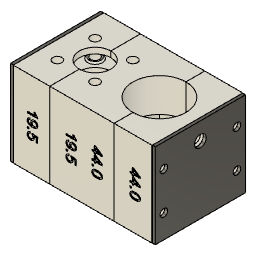
E39steerModuleCase v1 (Autodesk Fusion 360 design; units mm, degrees)
Autodesk Fusion 360 part; units mm, degrees
note: some values were not read from the file. Set by a fixed rule: which face or edge a step refers to.
sketch "Sketch1" plane through (0, 0, 0) normal (0, 0, 1) x (1, 0, 0)
  circle A0 centre (0, 0) radius 9.75
  line L0 (0, 0) -> (-27.3416, 27.3416) construction
  line L1 (0, 0) -> (-38.1238, 0) construction
  circle A1 centre (-12.9047, 12.9047) radius 9.3
  line L2 (0, 0) -> (-25, 0)
  line L3 (-25, 0) -> (-25, 31)
  line L4 (-25, 31) -> (0, 31)
  line L5 (0, 31) -> (0, 0)
  circle A2 centre (-12.9047, 12.9047) radius 3.1
  circle A3 centre (0, 0) radius 10.75
  circle A4 centre (-12.9047, 12.9047) radius 4
  line L6 (0, 31) -> (0, 19.6239) construction
  line L7 (-25, 0) -> (-19.6239, 0) construction
  circle A5 centre (-12.9047, 12.9047) radius 8.5 construction
  circle A6 centre (-12.9047, 12.9047) radius 2
  line L8 (-12.9047, 22.2047) -> (0, 22.2047)
  line L9 (-22.2047, 12.9047) -> (-22.2047, 0)
  dimension "d1" = 19.5
  dimension "d3" = 45
  dimension "d4" = 18.6
  dimension "d6" = 31
  dimension "d7" = 6.2
  dimension "d8" = 21.5
  dimension "d15" = 8
  dimension "d119" = 17
  dimension "d151" = 4
  dimension "d172" = 18.25
  dimension "d173" = 25
  constraint coincident A0.centre L0.start
  constraint horizontal L1
  constraint horizontal L2
  constraint vertical L3
  constraint horizontal L4
  constraint vertical L5
  constraint concentric A1 A2
  constraint concentric A2 A4
  constraint perpendicular L4 L6
  constraint perpendicular L3 L7
  constraint concentric A4 A5
  constraint concentric A2 A6
  constraint coincident A1 L8.start
  constraint coincident L5 L8.end
  constraint tangent A1 L8
  constraint perpendicular L5 L8
  constraint vertical L9
  constraint coincident A1 L9.start
  constraint coincident L1 L9.end
  measures "d1" diameter of A0
  measures "d3" angle of L0 L1
  measures "d4" diameter of A1
  measures "d6" distance of A0.centre L4.end
  measures "d7" diameter of A2
  measures "d8" diameter of A3
  measures "d15" diameter of A4
  measures "d119" diameter of A5
  measures "d151" diameter of A6
  measures "d172" distance of A0.centre A1.centre
  measures "d173" distance of L3.end L4.end
extrude "Extrude1" add sketch "Sketch1" along normal blind 16 contours A1 L5 A3 L8 | A1 L2 A3 L9 | A1 A3 | A1 L2 L3 L4 L5 L8 L9 | A2 | A4 | A6 makes body 1
extrude "Extrude3" cut sketch "Sketch1" along normal blind 12 contours A0 A1 | A0 A1 A3 | A1 L5 A3 L8 | A1 L2 A3 L9 | A1 A3 | A4 bodies 1
extrude "Extrude2" cut sketch "Sketch1" along normal blind 14 contours A2 | A6 bodies 1
extrude "Extrude4" cut sketch "Sketch1" along normal blind 13 contours A4 bodies 1
extrude "Extrude15" add 1 faces at (-9.2311, 12.552, 13) along direction (0, 0, -1) blind 2 on bodies 1 bodies 1
extrude "Extrude20" add sketch "Sketch1" along normal blind 4 contours A1 L5 A3 L8 | A1 L2 A3 L9 | A1 A3 | A1 L2 L3 L4 L5 L8 L9 bodies 1
extrude "Extrude21" add sketch "Sketch1" along normal blind 5 contours A4 bodies 1
extrude "Extrude31" cut sketch "Sketch1" along normal up to surface (16 mm away) contours A6 bodies 1
chamfer "Chamfer2" distance 1 angle 45 2 edges at (-16.634, 11.4582, 12) (-16.634, 14.3512, 4) on bodies 1
ref_plane "WorkPlane2" through (-12.5, 15.5, -13) normal (0, 0, -1) x (-1, 0, 0)
mirror "Mirror1" about plane through (-12.5, 15.5, -13) normal (0, 0, -1) of bodies 1 makes body 2
extrude "Extrude5" cut 1 faces at (-10.1904, 12.6513, -40) along direction (0, 0, -1) blind 3 on bodies 2 bodies 2
extrude "Extrude6" add sketch "Sketch1" 1 faces at (-12.5577, 25.9987, 0) along normal up to surface contours A1 L5 A3 L8 | A1 L2 A3 L9 | A1 A3 | A1 L2 L3 L4 L5 L8 L9 end surface through (0, 0, -26) normal (0, 0, 1) offset 0 on bodies 1 bodies 1 2
sketch "Sketch3" plane through (-25, 0, 0) normal (-1, 0, 0) x (0, -1, 0)
  line L0 (0, -42) -> (0, 16)
  line L1 (0, 16) -> (-31, 16)
  line L2 (-31, 16) -> (-9.7868, 16) construction
  line L3 (-31, 16) -> (-25, 16) construction
  line L4 (-25, 16) -> (-25, 0) construction
  circle A0 centre (-25, 0) radius 2.6
  line L5 (-31, 16) -> (-31, -42)
  line L6 (-31, -42) -> (0, -42)
  circle A1 centre (-25, -26) radius 2.6
  dimension "d27" = 6
  dimension "d28" = 16
  dimension "d29" = 5.2
  dimension "d178" = 5.2
  dimension "d179" = 26
  constraint horizontal L2
  constraint coincident L1.end L2.start
  constraint perpendicular L3 L4
  constraint coincident L4.end A0.centre
  measures "d27" distance of L1.end L3.end
  measures "d28" distance of L3.end L4.end
  measures "d29" diameter of A0
  measures "d178" diameter of A1
  measures "d179" distance of L4.end A1.centre
extrude "Extrude7" cut sketch "Sketch3" against normal up to surface (25 mm away) contours A0 | A1 bodies 1
sketch "Sketch10" plane through (0, 0, 0) normal (1, 0, 0) x (0, 1, 0)
  circle A0 centre (25, 0) radius 2.6
  line L0 (22.2047, 4) -> (10.75, 4)
  line L1 (10.75, 4) -> (10.75, -30)
  line L2 (10.75, -30) -> (22.2047, -30)
  line L3 (22.2047, -38) -> (10.75, -38)
  line L4 (10.75, -38) -> (10.75, -42)
  line L5 (10.75, -42) -> (31, -42)
  line L6 (31, -42) -> (31, 16)
  line L7 (31, 16) -> (10.75, 16)
  line L8 (10.75, 16) -> (10.75, 12)
  line L9 (10.75, 12) -> (22.2047, 12)
  line L10 (10.75, 4) -> (10.75, -9) construction
  line L11 (22.25, -9) -> (26.25, -9)
  line L12 (26.25, -9) -> (26.25, -17)
  line L13 (26.25, -17) -> (22.25, -17)
  line L14 (22.25, -17) -> (22.25, -9)
  circle A1 centre (25, -26) radius 2.6
  line L15 (22.2047, 12) -> (22.2047, 4)
  line L16 (22.2047, -30) -> (22.2047, -38)
  dimension "d136" = 11.5
  dimension "d137" = 4
  dimension "d138" = 8
  dimension "d180" = 25
  constraint coincident L0.end L1.start
  constraint perpendicular L0 L10
  constraint horizontal L11
  constraint vertical L12
  constraint horizontal L13
  constraint vertical L14
  measures "d136" distance of L10.end L11.start
  measures "d137" distance of L11.start L11.end
  measures "d138" distance of L11.start L13.end
  measures "d180" distance of L7 L11.end
extrude "Extrude26" add sketch "Sketch10" along normal blind 5 contours L11 L12 L13 L14 bodies 1
mirror "Mirror2" about plane through (-10.75, 0, 0) normal (0, -1, 0) of bodies 1 merged
mirror "Mirror3" about plane through (0, -22.2047, 0) normal (1, 0, 0) of bodies 1 makes body 3
move_face "OffsetFaces1" offset -0.1 8 faces at (1.6667, 23.5833, -9) (1.6667, 26.25, -11.6667) (3.3333, 22.25, -14.3333) (1.6667, 24.9167, -17) (1.6667, -26.25, -11.6667) (1.6667, -24.9167, -17) (3.3333, -22.25, -14.3333) (1.6667, -23.5833, -9) on bodies 1
sketch "Sketch5" plane through (0, 0, -42) normal (0, 0, -1) x (1, 0, 0)
  circle A0 centre (12.9047, 12.9047) radius 3.1
  line L0 (0, -31) -> (25, -31)
  line L1 (25, 31) -> (0, 31)
  line L2 (0, 31) -> (0, 10.75)
  arc A1 (0, -10.75) -> (0, 10.75) centre (0, 0) ccw
  line L3 (0, -10.75) -> (0, -31)
  line L4 (24, 30.9926) -> (24, 30.9994) construction
  circle A2 centre (44, -0.0006) radius 18.1
  circle A3 centre (12.9047, -12.9047) radius 3.1
  line L5 (65, -21.1006) -> (23, -21.1006)
  line L6 (23, -21.1006) -> (23, 21.0994)
  line L7 (23, 21.0994) -> (65, 21.0994)
  line L8 (65, 21.0994) -> (65, -21.1006)
  line L9 (65, -21.1006) -> (23, 21.0994) construction
  line L10 (23, -21.1006) -> (65, 21.0994) construction
  point P0 (24, 9.8926)
  point P1 (24, -0.0006)
  point P2 (44, -0.0006)
  dimension "d126" = 36.2
  dimension "d182" = 44
  dimension "d183" = 42
  dimension "d184" = 42.2
  constraint horizontal L5
  constraint perpendicular L5 L6
  constraint parallel L5 L7
  constraint parallel L6 L8
  constraint coincident L9 P2
  constraint coincident L10 P2
  constraint coincident P2 A2.centre
  measures "d126" diameter of A2
  measures "d182" horizontal distance of A1.centre P2
  measures "d183" distance of L6.end L7.end
  measures "d184" distance of L5.end L6.end
extrude "Extrude37" add 1 faces at (25, -7.5525, -16.9573) along direction (1, 0, 0) blind 45 on bodies 3 bodies 3
extrude "Extrude38" cut sketch "Sketch5" against normal up to surface (58 mm away) contours A2 | L5 L6 L7 L8 bodies 3
chamfer "Chamfer4" distance 6 angle 45 2 edges at (65, 21.1006, -13) (65, -21.0994, -13) on bodies 3
extrude "Extrude39" cut sketch "Sketch5" against normal blind 36.5 contours L5 L6 L7 L8 bodies 3
extrude "Extrude40" add sketch "Sketch5" against normal blind 23 contours L5 L6 L7 L8 bodies 3
ref_plane "WorkPlane1" through (44, 0.0006, -13) normal (1, 0, 0) x (0, 1, 0)
split "Split2" by plane through (44, 0.0006, -13) normal (1, 0, 0) bodies 3 makes body 4 at (70, -7.5525, -16.9573)
extrude "Extrude27" cut 2 faces at (-5, 23.5833, -14.3333) (-5, -23.5833, -14.3333) along direction (1, 0, 0) blind 50 on bodies 3 bodies 3 4
extrude "Extrude30" add 2 faces at (45, -23.5833, -14.3333) (45, 23.5833, -14.3333) along direction (-1, 0, 0) blind 6 on bodies 4 bodies 4
move_face "OffsetFaces2" offset -0.1 8 faces at (42.3333, 26.25, -11.6667) (42.3333, 24.9167, -17) (42.3333, -24.9167, -17) (42.3333, -22.25, -14.3333) (42.3333, -26.25, -11.6667) (42.3333, 22.25, -14.3333) (42.3333, 23.5833, -9) (42.3333, -23.5833, -9) on bodies 4
sketch "Sketch11" plane through (70, 0, 0) normal (1, 0, 0) x (0, 1, 0)
  line L0 (30, 16) -> (-29.9994, 16)
  circle A0 centre (-25, 4) radius 2.6
  circle A1 centre (25, 4) radius 2.6
  circle A2 centre (0, -30) radius 4
  line L1 (-3.7816, -23.45) -> (-7.5633, -30)
  line L2 (-7.5633, -30) -> (-3.7816, -36.55)
  line L3 (-3.7816, -36.55) -> (3.7816, -36.55)
  line L4 (3.7816, -36.55) -> (7.5633, -30)
  line L5 (7.5633, -30) -> (3.7816, -23.45)
  line L6 (3.7816, -23.45) -> (-3.7816, -23.45)
  circle A3 centre (-25, -26) radius 2.6
  circle A4 centre (-25, 0) radius 2.6
  circle A5 centre (25, 0) radius 2.6
  circle A6 centre (25, -26) radius 2.6
  line L7 (31, 16) -> (-31, 16)
  line L8 (-31, 16) -> (-31, -42)
  line L9 (-31, -42) -> (31, -42)
  line L10 (31, -42) -> (31, 16)
  point P0 (0, -30)
  dimension "d154" = 8
  dimension "d155" = 6.55
  dimension "d196" = 46
  constraint coincident P0 A2.centre
  measures "d154" diameter of A2
  measures "d155" distance of P0 L6
  measures "d196" distance of L0 P0
extrude "Extrude32" cut sketch "Sketch11" against normal up to surface (26 mm away) contours A2 | L1 L2 L3 L4 L5 L6 bodies 4
extrude "Extrude33" add sketch "Sketch11" against normal blind 2 contours L1 L2 L3 L4 L5 L6 bodies 4
fillet "Fillet3" radius 0.2 4 edges at (-25, -31, -13) (-25, 31, -13) (70, 31, -13) (70, -31, -13) on bodies 1 4
extrude "Extrude1'" add 1 faces at (70, 0.0996, -8.9287) along direction (1, 0, 0) blind 2 separate body on bodies 4 makes body 5 in component "Right Plate"
extrude "Extrude1''" add 1 faces at (-25, 7.5525, -16.9573) along direction (-1, 0, 0) blind 2 separate body on bodies 1 makes body 6 in component "Left Plate"
sketch "Sketch15" plane through (0, 31, 0) normal (0, 1, 0) x (-1, 0, 0)
  line L0 (24.8, -42) -> (24.8, 16)
  line L1 (24.8, 16) -> (0, 16)
  line L2 (0, 16) -> (0, -42)
  line L3 (0, -42) -> (24.8, -42)
  line L4 (16.897, -21.1711) -> (16.9507, -2.3279) construction
  line L5 (16.9507, -2.3279) -> (8.3674, -2.3034) construction
  line L6 (8.3674, -2.3034) -> (8.3137, -21.1466) construction
  line L7 (8.3137, -21.1466) -> (16.897, -21.1711) construction
  line L8 (16.897, -21.1711) -> (16.9507, -2.3279) construction
  line L9 (16.9507, -2.3279) -> (8.3674, -2.3034) construction
  line L10 (8.3674, -2.3034) -> (8.3137, -21.1466) construction
  line L11 (8.3137, -21.1466) -> (16.897, -21.1711) construction
  line L12 (-9.5874, -21.1711) -> (-9.5336, -2.3279) construction
  line L13 (-9.5336, -2.3279) -> (-18.117, -2.3034) construction
  line L14 (-18.117, -2.3034) -> (-18.1707, -21.1466) construction
  line L15 (-18.1707, -21.1466) -> (-9.5874, -21.1711) construction
  dimension "d358" = 7
  dimension "d361" = 7
  dimension "d362" = 7
  text T0 "19.5" font "Arial" height 7 align left top in box 18.8432 x 8.5834 at (16.897, -21.1711) x (0.002851, 0.999996) y (-0.999996, 0.002851) spacing 1 kerned
  text T1 "19.5" font "Arial" height 7 align left top in box 18.8432 x 8.5834 at (-9.5874, -21.1711) x (0.002851, 0.999996) y (-0.999996, 0.002851) spacing 1 kerned
extrude "Extrude42" cut sketch "Sketch15" 1 faces at (29.3333, 31, -22.6667) against normal blind 0.2 text T0 T1 on bodies 3 bodies 1
sketch "Sketch17" plane through (0, 31, 0) normal (0, 1, 0) x (-1, 0, 0)
  line L0 (-44, 16) -> (-44, -42)
  line L1 (-44, -42) -> (0, -42)
  line L2 (0, -42) -> (0, 16)
  line L3 (0, 16) -> (-44, 16)
  line L4 (-28.569, -22.0524) -> (-28.6455, -5.3707) construction
  line L5 (-28.6455, -5.3707) -> (-35.8666, -5.4038) construction
  line L6 (-35.8666, -5.4038) -> (-35.7901, -22.0855) construction
  line L7 (-35.7901, -22.0855) -> (-28.569, -22.0524) construction
  line L8 (-54.569, -22.0524) -> (-54.6455, -5.3707) construction
  line L9 (-54.6455, -5.3707) -> (-61.8666, -5.4038) construction
  line L10 (-61.8666, -5.4038) -> (-61.7901, -22.0855) construction
  line L11 (-61.7901, -22.0855) -> (-54.569, -22.0524) construction
  dimension "d363" = 7
  dimension "d366" = 7
  text T0 "44.0" font "Arial" height 7 align left top in box 16.6819 x 7.2212 at (-28.569, -22.0524) x (-0.004587, 0.999989) y (-0.999989, -0.004587) spacing 1 kerned
  text T1 "44.0" font "Arial" height 7 align left top in box 16.6819 x 7.2212 at (-54.569, -22.0524) x (-0.004587, 0.999989) y (-0.999989, -0.004587) spacing 1 kerned
extrude "Extrude43" cut sketch "Sketch17" sketch "Sketch15" against normal blind 0.2 text T0 of sketch 2 text T1 bodies 3
extrude "Extrude44" cut sketch "Sketch17" against normal blind 0.2 text T1 bodies 4
component "Right Plate" placed x (1, 0, 0) y (0, 1, 0) z (0, 0, 1) at (0, 0, 0)
component "Left Plate" placed x (1, 0, 0) y (0, 1, 0) z (0, 0, 1) at (0, 0, 0)
equation "d1 = SteerSaftDiameter"
equation "d4 = d119 + 1.6 mm"
equation "d6 = 25 mm + 6 mm"
equation "d8 = SteerSaftDiameter + 2 mm"
equation "d13 = 16 mm - BearingCaseWallThickness"
equation "d15 = 6 mm + ( ( 2 * 1 ) * 1 mm )"
equation "d16 = 16 mm - BearingCaseWallThickness + 1 mm"
equation "d28 = StubHoleDistanceEdge"
equation "d106 = d183 / 2"
equation "d107 = 14 mm - BearingCaseWallThickness - BearingWidth"
equation "d109 = 15 mm - BearingCaseWallThickness - BearingWidth"
equation "d119 = BearingDiameter"
equation "d124 = 2 * 42 mm"
equation "d141 = -GearDistance - 6 mm"
equation "d155 = ( 13.1 / 2 ) * 1 mm"
equation "SteerSaftDiameter = 19.5 mm" comment "What is the diameter of the steering shaft"
equation "BearingDiameter = 17 mm"
equation "CaseHeight = 58 mm" comment "Case height in Z-axis"
equation "StubHoleDistanceEdge = 16 mm" comment "Through hole connecting threaded rod distance from the case side"
equation "d172 = ( SteerSaftDiameter / 2 ) + ( BearingDiameter / 2 )"
equation "CaseQuarteDistance = ( CaseHeight - ( ( 16 * 2 ) * 1 mm ) ) / 2"
equation "d177 = CaseQuarteDistance"
equation "d178 = d29"
equation "d179 = CaseHeight - ( StubHoleDistanceEdge * 2 )"
equation "d180 = ( CaseHeight / 2 ) - ( d138 / 2 )"
equation "GearDistance = 44 mm" comment "Distance between gear saft center point and SSC motor center point"
equation "d182 = GearDistance"
equation "d185 = GearDistance - d173 + ( d183 / 2 ) + 5 mm"
equation "d190 = -CaseHeight + 35 mm - 13.5 mm"
equation "d192 = -CaseHeight + 35 mm"
equation "BoltCenterOffset = 17 mm" comment "Connecting rod bolt placement from center of the case (Z-axis), positive value will move the bolt placement closer to gearside of the case"
equation "BoltPosition = ( CaseHeight / 2 ) + BoltCenterOffset"
equation "d196 = BoltPosition"
equation "BearingWidth = 6 mm"
equation "BearingCaseWallThickness = 4 mm"
named bodies: "Body2", "Body3"
